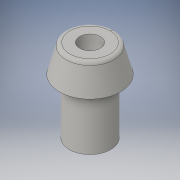
# Autodesk Inventor part: luer_fit
Saved by Autodesk Inventor 2016 (Build 200138000, 138)
## iProperties
Created: 2016-02-11
Part Number: luer_fit
Material: Generic
Document SubType Name: Modeling
Designer: GentnerLab
Density: 1 g/cm^3
Appearance: Default
Author: GentnerLab
Autodesk Inventor part; units mm, degrees
ref_plane "YZ Plane" through (0, 0, 0) normal (1, 0, 0) x (0, 1, 0)
ref_plane "XZ Plane" through (0, 0, 0) normal (0, 1, 0) x (-1, 0, 0)
ref_plane "XY Plane" through (0, 0, 0) normal (0, 0, 1) x (1, 0, 0)
sketch "Sketch1" plane through (0, 0, 0) normal (1, 0, 0) x (0, 1, 0)
  line L0 (0, -0.7937) -> (6.35, -0.7937)
  line L1 (6.35, -0.7937) -> (6.35, -1.7859)
  line L2 (6.35, -1.7859) -> (4.2333, -2.3531)
  line L3 (4.2333, -2.3531) -> (4.2333, -1.5875)
  line L4 (4.2333, -1.5875) -> (0, -1.5875)
  line L5 (0, -1.5875) -> (0, -0.7937)
  line L6 (0, -2.8237) -> (0, 0.4706) projected
  line L7 (-1.27, 0) -> (7.62, 0) projected
  point P0 (0, 0)
  dimension "d0" = 0.7937
  dimension "d1" = 6.35
  dimension "d2" = 4.2333
  dimension "d3" = 1.5875
  dimension "d4" = 0.9922
  dimension "d5" = 75
  constraints: 12 end point, 3 perpendicular, 1 horizontal, 1 parallel
  measures "d0" distance of L0.start point (0, 0)
  measures "d1" distance of L0.end L0.start
  measures "d2" distance of L4.end L3.end
  measures "d3" distance from line of point (0, 0) L4
  measures "d4" distance from line of L0 L1.end
  measures "d5" angle of L3 L2
revolve "Revolution1" add sketch "Sketch1" angle 360 about axis through (0, -10, 0) along (0, 1, 0)
fillet "Fillet1" radius 0.3175 1 edges at (0, 6.35, 1.7859) curvature continuous yes
equation "\"d2\" = 0.666667 * d1"
equation "\"d4\" = -1.25 * d0 + 1.25 * d3"
body "Solid1"
